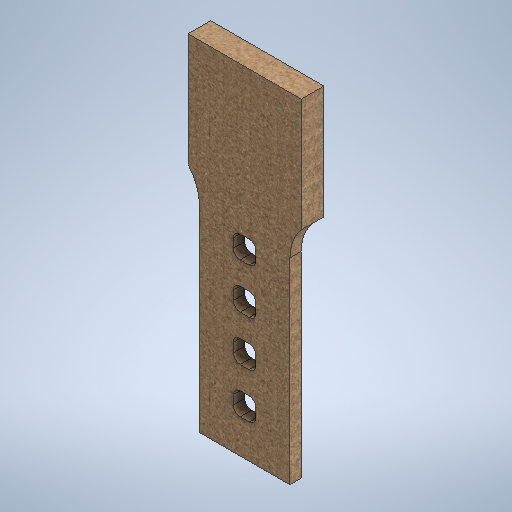
# Autodesk Inventor part: Pieza1
Saved by Autodesk Inventor 2025.3 (Build 293356000, 356)
## iProperties
Created: 2025-06-14
Part Number: Pieza1
Material: MDF Tablero de fibras de densidad media
Document SubType Name: Modeling
Designer: renato
Density: 0.8 g/cm^3
Appearance: Cartón - Ondulado
Mass: 34.8055 g
Surface Area: 158.139 cm^2
Volume: 43.5068 cm^3
Author: renato
Autodesk Inventor part; units mm, degrees
ref_plane "YZ Plane" through (0, 0, 0) normal (1, 0, 0) x (0, 1, 0)
ref_plane "XZ Plane" through (0, 0, 0) normal (0, 1, 0) x (-1, 0, 0)
ref_plane "XY Plane" through (0, 0, 0) normal (0, 0, 1) x (1, 0, 0)
sketch "Boceto1" plane through (0, 0, 0) normal (0, 0, 1) x (1, 0, 0)
  line L0 (-20, -50) -> (20, -50)
  line L1 (20, -50) -> (20, 50)
  line L2 (20, 50) -> (-20, 50)
  line L3 (-20, 50) -> (-20, -50)
  line L4 (-20, -50) -> (20, 50) construction
  line L5 (20, -50) -> (-20, 50) construction
  line L6 (-25, 100) -> (25, 100)
  line L7 (25, 100) -> (25, 50)
  line L8 (25, 50) -> (-25, 50)
  line L9 (-25, 50) -> (-25, 100)
  line L10 (-25, 100) -> (25, 50) construction
  line L11 (25, 100) -> (-25, 50) construction
  line L12 (-25, -50) -> (25, -50)
  line L13 (25, -50) -> (25, -100)
  line L14 (25, -100) -> (-25, -100)
  line L15 (-25, -100) -> (-25, -50)
  line L16 (-25, -50) -> (25, -100) construction
  line L17 (25, -50) -> (-25, -100) construction
  line L18 (0, 50) -> (0, 30) construction
  line L19 (0, 30) -> (0, 10) construction
  line L20 (0, 10) -> (0, -10) construction
  line L21 (0, -10) -> (0, -30) construction
  line L22 (0, -30) -> (0, -50) construction
  line L23 (0, 30) -> (0, 30) construction
  line L24 (0, 10) -> (0, 10) construction
  line L25 (0, -10) -> (0, -10) construction
  line L26 (0, -30) -> (0, -30) construction
  line L27 (2, 35) -> (-2, 35)
  line L28 (-5, 32) -> (-5, 28)
  line L29 (-2, 25) -> (2, 25)
  line L30 (5, 28) -> (5, 32)
  line L31 (5, 35) -> (-5, 25) construction
  line L32 (-5, 35) -> (5, 25) construction
  line L33 (2, 15) -> (-2, 15)
  line L34 (-5, 12) -> (-5, 8)
  line L35 (-2, 5) -> (2, 5)
  line L36 (5, 8) -> (5, 12)
  line L37 (5, 15) -> (-5, 5) construction
  line L38 (-5, 15) -> (5, 5) construction
  line L39 (2, -5) -> (-2, -5)
  line L40 (-5, -8) -> (-5, -12)
  line L41 (-2, -15) -> (2, -15)
  line L42 (5, -12) -> (5, -8)
  line L43 (5, -5) -> (-5, -15) construction
  line L44 (-5, -5) -> (5, -15) construction
  line L45 (2, -25) -> (-2, -25)
  line L46 (-5, -28) -> (-5, -32)
  line L47 (-2, -35) -> (2, -35)
  line L48 (5, -32) -> (5, -28)
  line L49 (5, -25) -> (-5, -35) construction
  line L50 (-5, -25) -> (5, -35) construction
  line L51 (0, 30) -> (0, 10) construction
  arc A0 (-2, 35) -> (-5, 32) centre (-2, 32) ccw
  arc A1 (5, 32) -> (2, 35) centre (2, 32) ccw
  arc A2 (2, 25) -> (5, 28) centre (2, 28) ccw
  arc A3 (-5, 28) -> (-2, 25) centre (-2, 28) ccw
  arc A4 (-2, 15) -> (-5, 12) centre (-2, 12) ccw
  arc A5 (-5, 8) -> (-2, 5) centre (-2, 8) ccw
  arc A6 (2, 5) -> (5, 8) centre (2, 8) ccw
  arc A7 (5, 12) -> (2, 15) centre (2, 12) ccw
  arc A8 (5, -8) -> (2, -5) centre (2, -8) ccw
  arc A9 (-2, -5) -> (-5, -8) centre (-2, -8) ccw
  arc A10 (-5, -12) -> (-2, -15) centre (-2, -12) ccw
  arc A11 (2, -15) -> (5, -12) centre (2, -12) ccw
  arc A12 (5, -28) -> (2, -25) centre (2, -28) ccw
  arc A13 (2, -35) -> (5, -32) centre (2, -32) ccw
  arc A14 (-5, -32) -> (-2, -35) centre (-2, -32) ccw
  arc A15 (-2, -25) -> (-5, -28) centre (-2, -28) ccw
  point P0 (0, 0)
  point P1 (0, 75)
  point P2 (0, -75)
  dimension "d0" = 40
  dimension "d1" = 100
  dimension "d2" = 50
  dimension "d3" = 50
  dimension "d4" = 50
  dimension "d5" = 50
  dimension "d6" = 20
  dimension "d7" = 20
  dimension "d8" = 20
  dimension "d9" = 20
  dimension "d10" = 0
  dimension "d11" = 0
  dimension "d12" = 0
  dimension "d13" = 0
  dimension "d25" = 10
  dimension "d26" = 10
  dimension "d27" = 10
  dimension "d28" = 10
  dimension "d29" = 10
  dimension "d30" = 10
  dimension "d31" = 10
  dimension "d32" = 10
  dimension "d33" = 20
  dimension "d34" = 3
  constraints: 104 end point, 35 point on line, 32 point on circle, 32 tangent, 16 centre point, 15 equal length, 15 equal radius, 15 midpoint, 11 horizontal, 7 perpendicular, 1 vertical
  measures "d0" distance of L2.end L1.end
  measures "d1" distance of L1.end L0.end
  measures "d2" distance of L7.end L8.end
  measures "d3" distance of L6.end L7.end
  measures "d4" distance of L13.end L14.end
  measures "d5" distance of L12.end L13.end
  measures "d6" distance of L18.start L18.end
  measures "d7" distance of L18.end L19.end
  measures "d8" distance of L20.end L19.end
  measures "d9" distance of L20.end L21.end
  measures "d10" distance of L24.end L19.end
  measures "d11" distance of L20.end L25.end
  measures "d12" distance of L21.end L26.end
  measures "d13" distance of L18.end L23.end
  measures "d25" distance of L32.end L31.end
  measures "d26" distance of L31.end L32.start
  measures "d27" distance of L38.end L37.end
  measures "d28" distance of L37.end L38.start
  measures "d29" distance of L44.end L43.end
  measures "d30" distance of L43.end L44.start
  measures "d31" distance of L50.end L49.end
  measures "d32" distance of L49.end L50.start
  measures "d33" distance of L24.end L23.end
  measures "d34" radius of A0
extrude "Extrusión1" add sketch "Boceto1" along normal blind 10 contours L3 L2 L1 L0 | L8 L9 L6 L7 L2
extrude "Extrusión2" cut sketch "Boceto1" along normal blind 5 contours L3 L2 L1 L0 | A1 L30 A2 L29 A3 L28 A0 L27 | A7 L36 A6 L35 A5 L34 A4 L33 | A8 L42 A11 L41 A10 L40 A9 L39 | A12 L48 A13 L47 A14 L46 A15 L45
fillet "Empalme3" radius 20 2 edges at (20, 50, 7.5) (-20, 50, 7.5)
